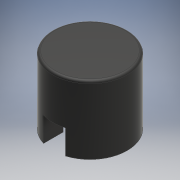
# Autodesk Inventor part: 48-0077
Saved by Autodesk Inventor 2018 (Build 220112000, 112)
## iProperties
Created: 2019-09-25
Part Number: 48-0077
Material: ABS Plastic
Document SubType Name: Modeling
Designer: Bradley
Density: 1.06 g/cm^3
Appearance: Smooth - Black
Author: Bradley
Autodesk Inventor part; units mm, degrees
ref_plane "YZ Plane" through (0, 0, 0) normal (1, 0, 0) x (0, 1, 0)
ref_plane "XZ Plane" through (0, 0, 0) normal (0, 1, 0) x (-1, 0, 0)
ref_plane "XY Plane" through (0, 0, 0) normal (0, 0, 1) x (1, 0, 0)
sketch "Sketch1" plane through (0, 0, 0) normal (0, 0, 1) x (1, 0, 0)
  circle A0 centre (0, 0) radius 3
  dimension "d0" = 6
  constraints: 1 centre point, 1 coincident
  measures "d0" diameter of A0
extrude "Extrusion1" add sketch "Sketch1" along normal mid plane 5.5
fillet "Fillet1" radius 0.2 1 edges at (-3, 0, 2.75)
fillet "Fillet1" radius 0.05 1 edges at (-3, 0, -2.75)
sketch "Sketch2" plane through (0, 0, -2.75) normal (0, 0, -1) x (-1, 0, 0)
  line L0 (1.25, -1.25) -> (-1.25, -1.25)
  line L1 (-1.25, -1.25) -> (-1.25, 1.25)
  line L2 (-1.25, 1.25) -> (1.25, 1.25)
  line L3 (1.25, 1.25) -> (1.25, -1.25)
  line L4 (1.25, -1.25) -> (-1.25, 1.25) construction
  line L5 (-1.25, -1.25) -> (1.25, 1.25) construction
  point P0 (0, 0)
  dimension "d5" = 2.5
  constraints: 12 end point, 2 midpoint, 2 parallel, 2 perpendicular, 1 horizontal
  measures "d5" distance of L1.end L2.end
extrude "Extrusion2" cut sketch "Sketch2" against normal blind 2.8
sketch "Sketch3" plane through (0, 0, -2.75) normal (0, 0, -1) x (-1, 0, 0)
  circle A0 centre (0, 0) radius 3 projected
  line L0 (-0.9, -3) -> (0.9, -3)
  line L1 (0.9, -3) -> (0.9, 3)
  line L2 (0.9, 3) -> (-0.9, 3)
  line L3 (-0.9, 3) -> (-0.9, -3)
  point P0 (0, 3)
  dimension "d8" = 1.8
  constraints: 8 end point, 2 parallel, 2 tangent, 1 horizontal, 1 midpoint, 1 perpendicular, 1 vertical alignment
  measures "d8" distance of L0.start L0.end
extrude "Extrusion3" cut sketch "Sketch3" against normal blind 2 contours L1 A0 L3 | A0 L2 L1 | L1 L0 A0 | A0 L3 L2 | L0 L3 A0
body "Solid1"
